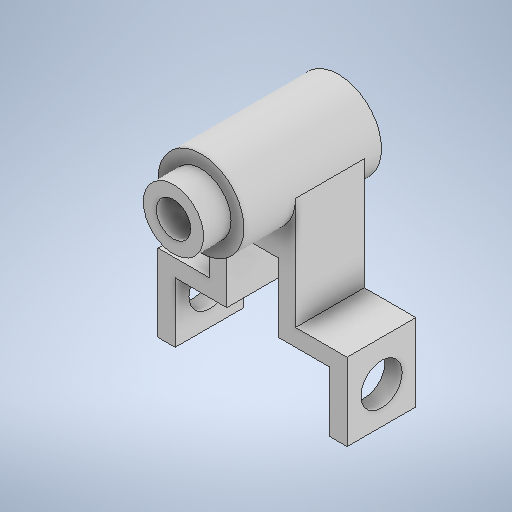
# Autodesk Inventor part: cad@54
Saved by Autodesk Inventor 2025.2 (Build 292293000, 293)
## iProperties
Created: 2025-04-09
Part Number: cad@54
Material: Generic
Document SubType Name: Modeling
Designer: spars
Density: 1 g/cm^3
Appearance: Default
Author: spars
Autodesk Inventor part; units mm, degrees
ref_plane "YZ Plane" through (0, 0, 0) normal (1, 0, 0) x (0, 1, 0)
ref_plane "XZ Plane" through (0, 0, 0) normal (0, 1, 0) x (-1, 0, 0)
ref_plane "XY Plane" through (0, 0, 0) normal (0, 0, 1) x (1, 0, 0)
sketch "Sketch1" plane through (0, 0, 0) normal (0, 0, 1) x (1, 0, 0)
  line L0 (-346.0753, 70.9014) -> (-181.3844, 70.9014) construction
  line L1 (-181.3844, 70.9014) -> (-181.3844, -72.4094) construction
  line L2 (-181.3844, -72.4094) -> (-346.0753, -72.4094) construction
  line L3 (-346.0753, -72.4094) -> (-346.0753, 70.9014) construction
  line L4 (25, 32.5) -> (25, -32.5)
  line L5 (-25, -32.5) -> (-25, 32.5)
  line L6 (-25, 32.5) -> (25, -32.5) construction
  line L7 (25, 32.5) -> (-25, -32.5) construction
  line L8 (15, -2.5) -> (-15, -2.5)
  arc A0 (-25, 32.5) -> (25, 32.5) centre (0, 32.5) ccw
  line L9 (-25, -32.5) -> (-55, -32.5)
  line L10 (-55, -32.5) -> (-55, -77.5)
  line L11 (-55, -77.5) -> (-45, -77.5)
  line L12 (-45, -77.5) -> (-45, -42.5)
  line L13 (25, -32.5) -> (55, -32.5)
  line L14 (55, -32.5) -> (55, -77.5)
  line L15 (55, -77.5) -> (45, -77.5)
  line L16 (45, -77.5) -> (45, -42.5)
  line L17 (-15, -2.5) -> (-15, -42.5)
  line L18 (15, -2.5) -> (15, -42.5)
  line L19 (-45, -42.5) -> (-15, -42.5)
  line L20 (15, -42.5) -> (45, -42.5)
  point P0 (0, 0)
  dimension "d3" = 50
  dimension "d4" = 65
  dimension "d15" = 25
  dimension "d16" = 90
  dimension "d18" = 30
  dimension "d19" = 45
  constraints: 34 end point, 7 perpendicular, 3 parallel, 2 horizontal, 2 midpoint, 2 point on circle, 1 centre point, 2 other
  measures "d3" distance of L4.end L5.start
  measures "d4" distance of L4.start L4.end
  measures "d15" radius of A0
  measures "d16" distance of L12.end L16.end
  measures "d18" distance of L5.start L9.end
  measures "d19" distance of L9.end L10.end
extrude "Extrusion1" add sketch "Sketch1" along normal blind 40
sketch "Sketch2" plane through (0, 0, 40) normal (0, 0, 1) x (1, 0, 0)
  arc A0 (-25, 32.5) -> (25, 32.5) centre (0, 32.5) ccw projected
  circle A1 centre (0, 32.5) radius 25
  point P0 (0, 0)
  point P1 (25, 32.5)
  dimension "d26" = 50
  constraints: 1 centre point, 1 coincident
  measures "d26" diameter of A1
extrude "Extrusion2" add sketch "Sketch2" along normal blind 30 and the other way blind 50
sketch "Sketch3" plane through (0, 32.5, 70) normal (0, 0, 1) x (1, 0, 0)
  arc A0 (-25, 0) -> (25, 0) centre (0, 0) ccw projected
  circle A1 centre (0, 0) radius 17.5
  circle A2 centre (0, 0) radius 10
  point P0 (0, -32.5)
  dimension "d31" = 35
  dimension "d32" = 20
  constraints: 2 centre point, 2 coincident
  measures "d31" diameter of A1
  measures "d32" diameter of A2
extrude "Extrusion3" add sketch "Sketch3" along normal blind 16
sketch "Sketch4" plane through (45, -77.5, 0) normal (0, -1, 0) x (1, 0, 0)
  point P0 (-45, 0)
sketch "Sketch5" plane through (55, -77.5, 0) normal (1, 0, 0) x (0, 0, -1)
  circle A0 centre (-20, 21.3987) radius 12
  line L0 (0, 0) -> (0, 45) projected
  point P0 (0, 77.5)
  dimension "d35" = 24
  dimension "d36" = 20
  constraints: 1 centre point
  measures "d35" diameter of A0
  measures "d36" distance from line of L0 A0.centre
extrude "Extrusion4" cut sketch "Sketch5" against normal blind 120
body "Solid1"
